61488eee-7316-4021-a618-65146cc97edb (Autodesk Fusion 360 design; units mm, degrees)
Autodesk Fusion 360 part; units mm, degrees
sketch "Sketch2" plane through (0, 0, 0) normal (1, 0, 0) x (0, 1, 0)
  line L0 (0, 0) -> (13.4874, 0) construction
  line L1 (27.3812, 0) -> (13.4874, 0) construction
  circle A0 centre (20.4343, 0) radius 6.9469
  dimension "d1" = 13.4874
  dimension "d2" = 27.3812
  constraint coincident L0.start origin
  constraint horizontal L0
  constraint parallel L0 L1
  constraint midpoint L1 A0.centre
  constraint coincident L1.start A0
  measures "d1" distance of L0.start L0.end
  measures "d2" distance of L0.start L1.start
revolve "Revolve4" add sketch "Sketch2" angle 360 about axis through (0, 0, 1.75) along (0, 0, 1) makes body 1
ref_plane "WorkPlane1" through (-27.3812, 0, 0) normal (1, 0, 0) x (0, 1, 0)
ref_plane "WorkPlane2" through (67.8688, 0, 0) normal (1, 0, 0) x (0, 1, 0)
ref_plane "WorkPlane3" through (32.9438, 0, 0) normal (1, 0, 0) x (0, 1, 0)
sketch "Sketch6" plane through (32.9438, 0, 0) normal (1, 0, 0) x (0, 1, 0)
  circle A0 centre (0, 0) radius 5.5563
  dimension "d31" = 11.1125
  constraint coincident A0.centre origin
  measures "d31" diameter of A0
extrude "Extrude1" add sketch "Sketch6" along normal up to surface (34.925 mm away) separate body makes body 2
ref_plane "WorkPlane4" through (20.4343, 0, 0) normal (1, 0, 0) x (0, 1, 0)
sketch "Sketch7" plane through (0, 0, 0) normal (0, 0, 1) x (1, 0, 0)
  line L0 (20.4343, 0.75) -> (20.4343, 21.75)
  line L1 (0, 0) -> (76.2, 0) construction
  line L2 (20.4343, 18.7283) -> (20.4343, -25.4) construction
  line L3 (20.4343, 0) -> (37.1031, 0)
  line L4 (37.1031, 0) -> (37.1031, 9.8452)
  line L5 (20.4343, 0) -> (20.4343, 5.5563)
  line L6 (33.9407, 11.8592) -> (20.4343, 5.5562)
  arc A0 (37.1031, 9.8452) -> (33.9407, 11.8592) centre (34.8806, 9.8452) ccw
  point P0 (37.1031, 13.335)
  dimension "d40" = 16.6687
  dimension "d41" = 13.335
  dimension "d42" = 5.5563
  dimension "d43" = 2.2225
  constraint coincident L1.start origin
  constraint horizontal L1
  constraint coincident L0 L2.start
  constraint parallel L0 L2
  constraint coincident L2 L3.start
  constraint coincident L1 L3.start
  constraint perpendicular L2 L3
  constraint perpendicular L3 L4
  constraint perpendicular L3 L5
  constraint coincident P0 L4
  constraint coincident P0 L6
  constraint tangent L4 A0
  constraint tangent L6 A0
  measures "d40" distance of L3.start L3.end
  measures "d41" distance of L3.end P0
  measures "d42" distance of L3.start L5.end
  measures "d43" radius of A0
revolve "Revolve5" add sketch "Sketch7" angle 360 about axis through (0, 0, 0) along (1, 0, 0) bodies 1 2
thread "Thread2" "ANSI Unified Screw Threads 0.3125 5/16-18 UNC 3A" major diameter 7.8283 minor diameter 6.2586 pitch 1.4111 angle 60 modelled right hand crest width 0.2172 on face at (47.3583, 5.4843, 0.8913) crest through (36.7503, 3.9141, 0) on bodies 1
fillet "Fillet2" radius 2.2225 1 edges at (26.0703, -8.1231, -1.0178) on bodies 1
equation "d27 = -d2"
equation "d28 = 3.750 in"
equation "d30 = -1.375 in"
equation "EyeInner = d1"
equation "EyeOuter = d2"
equation "ThreadDia = d31"
equation "TotalLength = d28"
equation "ShankLength = d30"
equation "d39 = d1 + ( ( d2 - d1 ) ) / 2"
equation "d40 = d31 * 1.5"
equation "d41 = d31 * 1.2"
equation "d42 = d31 / 2"
equation "d43 = d31 * 0.2"
equation "d45 = d31 * 0.2"
